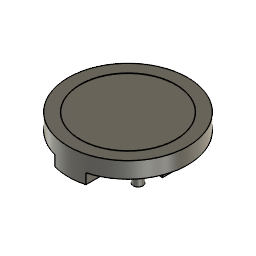
display stub (Autodesk Fusion 360 design; units mm, degrees)
Autodesk Fusion 360 part; units mm, degrees
sketch "Sketch1" plane through (0, 0, 0) normal (0, 0, 1) x (1, 0, 0)
  circle A0 centre (0, 0) radius 23
  dimension "d1" = 46
  constraint coincident A0.centre origin
  measures "d1" diameter of A0
extrude "Extrude1" add sketch "Sketch1" along normal blind 10.2
sketch "Sketch2" plane through (0, 0, 0) normal (0, 0, 1) x (1, 0, 0)
  line L0 (-16.25, 4.6) -> (-14.6, 4.6)
  line L1 (-14.6, 4.6) -> (-17.9, 4.6)
  line L2 (-17.9, 4.6) -> (-17.9, -4.6)
  line L3 (-17.9, -4.6) -> (-14.6, -4.6)
  line L4 (-14.6, -4.6) -> (-14.6, 4.6)
  line L5 (14.6, 0) -> (14.6, 4.6)
  line L6 (14.6, 4.6) -> (17.9, 4.6)
  line L7 (17.9, 4.6) -> (14.6, 4.6)
  line L8 (14.6, 4.6) -> (14.6, -4.6)
  line L9 (14.6, -4.6) -> (17.9, -4.6)
  line L10 (17.9, -4.6) -> (17.9, 4.6)
  dimension "d6" = 1.65
  dimension "d7" = 3.3
  dimension "d8" = 9.2
  dimension "d10" = 14.6
  dimension "d11" = 3.3
  dimension "d12" = 3.3
  dimension "d13" = 9.2
  constraint horizontal L1
  constraint vertical L2
  constraint horizontal L3
  constraint vertical L4
  constraint perpendicular L0 L5
  constraint perpendicular L5 L6
  constraint horizontal L7
  constraint vertical L8
  constraint horizontal L9
  constraint vertical L10
  measures "d6" distance of L0.start L0.end
  measures "d7" distance of L0.end L1.end
  measures "d8" distance of L0.end L3.end
  measures "d10" distance of origin L5.start
  measures "d11" distance of L5.end L6.end
  measures "d12" distance of L6.end L5.end
  measures "d13" distance of L6.end L9.end
extrude "Extrude2" add sketch "Sketch2" against normal blind 0.3
sketch "Sketch5" plane through (0, 0, 0) normal (0, 0, -1) x (1, 0, 0)
  line L0 (-14.6, -4.6) -> (-17.9, -4.6)
  line L1 (-17.9, -4.6) -> (-17.9, 4.6)
  line L2 (-17.9, 4.6) -> (-14.6, 4.6)
  line L3 (-14.6, 4.6) -> (-14.6, -4.6)
  line L4 (17.9, -4.6) -> (14.6, -4.6)
  line L5 (14.6, -4.6) -> (14.6, 4.6)
  line L6 (14.6, 4.6) -> (17.9, 4.6)
  line L7 (17.9, 4.6) -> (17.9, -4.6)
  circle A0 centre (0, 0) radius 23
  circle A1 centre (0, 0) radius 23
  line L8 (-17.9, 4.6) -> (-14.6, 4.6)
  line L9 (-14.6, 4.6) -> (-14.6, -4.6)
  line L10 (-14.6, -4.6) -> (-17.9, -4.6)
  line L11 (-17.9, -4.6) -> (-17.9, 4.6)
  line L12 (14.6, 4.6) -> (17.9, 4.6)
  line L13 (17.9, 4.6) -> (17.9, -4.6)
  line L14 (17.9, -4.6) -> (14.6, -4.6)
  line L15 (14.6, -4.6) -> (14.6, 4.6)
  constraint concentric A0 A1
  constraint horizontal L8
  constraint vertical L9
  constraint horizontal L10
  constraint vertical L11
  constraint coincident L0.start L3.end
  constraint coincident L1.end L2.start
  constraint horizontal L12
  constraint vertical L13
  constraint horizontal L14
  constraint vertical L15
  constraint coincident L4.start L7.end
  constraint coincident L5.end L6.start
extrude "Extrude3" cut 1 faces at (-0.5729, -10.7119, 0) along direction (0, 0, 1) blind 4
sketch "Sketch6" plane through (0, 0, 4) normal (0, 0, -1) x (1, 0, 0)
  line L0 (-14.6, -4.6) -> (-17.9, -4.6)
  line L1 (-17.9, -4.6) -> (-17.9, 4.6)
  line L2 (-17.9, 4.6) -> (-14.6, 4.6)
  line L3 (-14.6, 4.6) -> (-14.6, -4.6)
  line L4 (17.9, -4.6) -> (14.6, -4.6)
  line L5 (14.6, -4.6) -> (14.6, 4.6)
  line L6 (14.6, 4.6) -> (17.9, 4.6)
  line L7 (17.9, 4.6) -> (17.9, -4.6)
  circle A0 centre (0, 0) radius 23
  line L8 (0, 0) -> (0, 11.6)
  line L9 (0, 0) -> (0, -11.5)
  line L10 (0, 11.6) -> (-15.75, 11.6)
  line L11 (0, 11.6) -> (15.75, 11.6)
  line L12 (0, -11.5) -> (15.75, -11.5)
  line L13 (0, -11.5) -> (-15.75, -11.5)
  circle A1 centre (-15.75, 11.6) radius 1.9
  circle A2 centre (15.4643, 11.6) radius 1.9
  circle A3 centre (-15.75, -11.5) radius 1.9
  circle A4 centre (15.75, -11.5) radius 1.9
  dimension "d18" = 11.6
  dimension "d19" = 11.5
  dimension "d20" = 15.75
  dimension "d21" = 15.75
  dimension "d22" = 15.75
  dimension "d23" = 15.75
  dimension "d24" = 3.8
  dimension "d25" = 3.8
  dimension "d26" = 3.8
  dimension "d27" = 3.8
  constraint coincident A0.centre L8.start
  constraint vertical L8
  constraint vertical L9
  constraint perpendicular L8 L10
  constraint perpendicular L8 L11
  constraint perpendicular L9 L12
  constraint perpendicular L9 L13
  constraint coincident L10.end A1.centre
  constraint coincident L11 A2.centre
  constraint coincident L13.end A3.centre
  constraint coincident L12.end A4.centre
  measures "d18" distance of A0.centre L8.end
  measures "d19" distance of A0.centre L9.end
  measures "d20" distance of L8.end L10.end
  measures "d21" distance of L8.end L11.end
  measures "d22" distance of L9.end L12.end
  measures "d23" distance of L9.end L13.end
  measures "d24" diameter of A1
  measures "d25" diameter of A2
  measures "d26" diameter of A3
  measures "d27" diameter of A4
extrude "Extrude4" add sketch "Sketch6" along normal blind 4 contours A1 | A2 | A3 | A4
extrude "Extrude5" add 2 faces at (-15.7, -1.5333, -0.3) (15.7, 1.5333, -0.3) along direction (0, 0, -1) blind 0.2
sketch "Sketch7" plane through (0, 0, 0) normal (0, 1, 0) x (1, 0, 0)
sketch "Sketch8" plane through (0, 0, 0) normal (0, 0, 1) x (1, 0, 0)
  line L0 (0, 0) -> (15, 0)
  line L1 (15, 0) -> (15, 15.5)
  line L2 (15, 15.5) -> (0, 15.5)
  line L3 (0, 15.5) -> (0, 0)
  dimension "d32" = 15
  dimension "d33" = 15.5
  constraint horizontal L0
  constraint vertical L1
  constraint horizontal L2
  constraint vertical L3
  constraint coincident L0.start L3.end
  measures "d32" distance of L0.start L0.end
  measures "d33" distance of L0.start L2.end
sketch "Sketch9" plane through (0, 0, -0.5) normal (0, 0, -1) x (1, 0, 0)
  line L0 (17.9, -4.6) -> (17.9, 4.6)
  line L1 (17.9, 4.6) -> (14.6, 4.6)
  line L2 (14.6, 4.6) -> (14.6, -4.6)
  line L3 (14.6, -4.6) -> (17.9, -4.6)
  line L4 (15, -15.5) -> (-15, -15.5)
  line L5 (-15, -15.5) -> (-15, 15.5)
  line L6 (-15, 15.5) -> (15, 15.5)
  line L7 (15, 15.5) -> (15, -15.5)
  line L8 (0, 0) -> (16, 0)
  dimension "d34" = 30
  dimension "d35" = 31
  constraint horizontal L4
  constraint vertical L5
  constraint horizontal L6
  constraint vertical L7
  constraint horizontal L8
  measures "d34" distance of L4.start L4.end
  measures "d35" distance of L4.start L6.end
sketch "Sketch10" plane through (0, 0, 0) normal (0, 0, 1) x (1, 0, 0)
  line L0 (0, -23) -> (6, -23)
  line L1 (6, -23) -> (6, -14)
  line L2 (6, -14) -> (0, -14)
  line L3 (0, -14) -> (0, -23)
  line L4 (6, -14) -> (-6, -14)
  line L5 (-6, -14) -> (-6, -23)
  line L6 (-6, -23) -> (6, -23)
  line L7 (6, -23) -> (6, -14)
  circle A0 centre (0, 0) radius 23
  dimension "d36" = 6
  dimension "d37" = 12
  constraint horizontal L0
  constraint vertical L1
  constraint horizontal L2
  constraint vertical L3
  constraint horizontal L4
  constraint vertical L5
  constraint horizontal L6
  constraint vertical L7
  constraint coincident A0.centre origin
  constraint coincident L0.start A0
  constraint tangent L0 A0
  measures "d36" distance of L0.start L0.end
  measures "d37" distance of L1.end L4.end
extrude "Extrude6" add sketch "Sketch10" along normal blind 4 contours L3 L4 L5 A0 | L1 L2 L3 L4 L7 A0
sketch "Sketch11" plane through (0, 0, -0.5) normal (0, 0, -1) x (1, 0, 0)
  line L0 (0, 23) -> (0, 15.5)
  constraint vertical L0
sketch "Sketch12" plane through (0, 0, 0) normal (1, 0, 0) x (0, 1, 0)
sketch "Sketch13" plane through (0, 0, -0.5) normal (0, 0, -1) x (1, 0, 0)
  line L0 (0, 0) -> (-14.6, 0)
  line L1 (-14.6, 0) -> (-17.9, 0)
  line L2 (-14.6, 4.6) -> (-17.9, 4.6)
  line L3 (-17.9, 4.6) -> (-17.9, -4.6)
  line L4 (-17.9, -4.6) -> (-14.6, -4.6)
  line L5 (-14.6, -4.6) -> (-14.6, 4.6)
  constraint coincident L0.start origin
  constraint horizontal L0
  constraint parallel L0 L1
  constraint horizontal L2
  constraint vertical L3
  constraint horizontal L4
  constraint vertical L5
sketch "Sketch14" plane through (17.9, 0, 0) normal (1, 0, 0) x (0, 1, 0)
  line L0 (-4.6, 4) -> (-4.6, -0.5)
  line L1 (-4.6, -0.5) -> (4.6, -0.5)
  line L2 (4.6, -0.5) -> (4.6, 4)
  line L3 (4.6, 4) -> (-4.6, 4)
ref_plane "WorkPlane1" through (0, 0, 0) normal (1, 0, 0) x (0, 1, 0)
ref_plane "WorkPlane2" through (0, 0, 0) normal (0, 1, 0) x (0, 0, 1)
sketch "Sketch15" plane through (0, 0, 10.2) normal (0, 0, 1) x (-1, 0, 0)
  circle A0 centre (0, 0) radius 23
  circle A1 centre (0, 0) radius 18.375
  dimension "d42" = 36.75
  constraint coincident A0.centre A1.centre
  measures "d42" diameter of A1
extrude "Extrude7" cut sketch "Sketch15" against normal blind 0.1 contours A1
equation "d6 = ( 3.3 / 2 ) * 1 mm"
equation "d20 = ( 31.5 / 2 ) * 1 mm"
equation "d21 = ( 31.5 / 2 ) * 1 mm"
equation "d22 = ( 31.5 / 2 ) * 1 mm"
equation "d23 = ( 31.5 / 2 ) * 1 mm"
